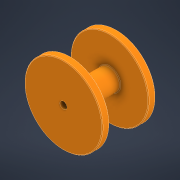
# Autodesk Inventor part: bushing_smConnection
Saved by Autodesk Inventor 2021 (Build 250183000, 183)
## iProperties
Created: 2021-06-22
Part Number: bushing_smConnection
Material: Generic
Document SubType Name: Modeling
Designer: Watchdog
Density: 1 g/cm^3
Appearance: Orange
Author: Watchdog
Autodesk Inventor part; units mm, degrees
ref_plane "YZ Plane" through (0, 0, 0) normal (1, 0, 0) x (0, 1, 0)
ref_plane "XZ Plane" through (0, 0, 0) normal (0, 1, 0) x (-1, 0, 0)
ref_plane "XY Plane" through (0, 0, 0) normal (0, 0, 1) x (1, 0, 0)
sketch "Sketch1" plane through (0, 0, 0) normal (0, 1, 0) x (-1, 0, 0)
  line L0 (110, -75) -> (10, -75)
  line L1 (10, 75) -> (110, 75)
  line L2 (110, 75) -> (110, 55)
  line L3 (110, 55) -> (30, 55)
  line L4 (30, 55) -> (30, -55)
  line L5 (30, -55) -> (110, -55)
  line L6 (110, -55) -> (110, -75)
  line L7 (0, 147.0752) -> (0, -168.5589)
  line L8 (10, 75) -> (10, -75)
  point P0 (0, 0)
  dimension "d6" = 20
  dimension "d7" = 20
  dimension "d10" = 55
  dimension "d11" = 110
  dimension "d15" = 10
  dimension "d16" = 30
  dimension "d17" = 110
  dimension "d18" = 110
  constraints: 18 end point, 4 perpendicular, 1 horizontal, 1 parallel, 1 point on line, 1 vertical
  measures "d6" distance between parallel lines of L0 L5
  measures "d7" distance between parallel lines of L1 L3
  measures "d10" distance from line of point (0, 0) L5
  measures "d11" distance between parallel lines of L3 L5
  measures "d15" horizontal distance of L7.end L0.end
  measures "d16" distance from line of point (0, 0) L4
  measures "d17" horizontal distance of L7.end L0.start
  measures "d18" horizontal distance of L7.end L1.end
revolve "Revolution1" add sketch "Sketch1" angle 360 about axis through (0, 0, 147.0752) along (0, 0, -1)
fillet "Fillet1" radius 2 2 edges at (30, 0, -55) (30, 0, 55)
fillet "Fillet2" radius 2 4 edges at (110, 0, 55) (110, 0, 75) (110, 0, -55) (110, 0, -75)
equation "\"d7\" = d6"
equation "\"d10\" = 0.5 * d11"
equation "\"d18\" = d17"
body "Solid1"
